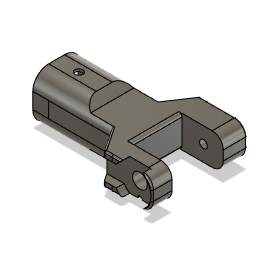
SholderFork_1 v20 (Autodesk Fusion 360 design; units mm, degrees)
Autodesk Fusion 360 part; units mm, degrees
note: some values were not read from the file. Chosen so that the rebuilt part matches the saved one: which face or edge a step refers to. Set by a fixed rule: which sketch regions a step uses.
sketch "Sketch1" plane through (0, 0, 0) normal (0, 1, 0) x (1, 0, 0)
  line L0 (-50, -15) -> (-10, -15)
  line L1 (-50, 15) -> (-10, 15)
  line L2 (5, -15) -> (5, 15)
  line L3 (30, 30) -> (5, 30)
  line L4 (30, -30) -> (5, -30)
  line L5 (5, -15) -> (30, -15)
  line L6 (30, -15) -> (30, -30)
  line L7 (5, 15) -> (30, 15)
  line L8 (30, 15) -> (30, 30)
  line L9 (-10, -15) -> (0, -30)
  line L10 (0, -30) -> (5, -30)
  line L11 (-10, 15) -> (0, 30)
  line L12 (0, 30) -> (5, 30)
  line L13 (-10, 15) -> (-10, -15)
  line L14 (-50, 15) -> (-60, 15)
  line L15 (-60, 15) -> (-60, -15)
  line L16 (-60, -15) -> (-50, -15)
  constraint horizontal L3
  constraint perpendicular L2 L5
  constraint perpendicular L4 L6
  constraint perpendicular L2 L7
  constraint perpendicular L3 L8
  constraint perpendicular L0 L13
  constraint perpendicular L14 L15
extrude "Extrude1" add sketch "Sketch1" along normal blind 30 makes body 1
sketch "Sketch3" plane through (-60, 0, 0) normal (-1, 0, 0) x (0, 0, 1)
  line L0 (-15, 0) -> (15, 0)
  line L1 (15, 0) -> (15, 30)
  line L2 (15, 30) -> (-15, 30)
  line L3 (-15, 30) -> (-15, 0)
  circle A0 through (13.6, 15, 10) (-6.8, 26.7779, 10) (-6.8, 3.2221, 10)
  line L4 (-15, 0) -> (15, 0)
  line L5 (15, 0) -> (15, 30)
  line L6 (15, 30) -> (-15, 30)
  line L7 (-15, 30) -> (-15, 0)
  dimension "d64" = 27.2
sketch "Sketch3 (curves 10 mm off its plane)" plane through (-70, 0, 0) normal (-1, 0, 0) x (0, 0, 1)
  circle A0 centre (0, 15) radius 13.6
extrude "Extrude3" cut sketch "Sketch3 (curves 10 mm off its plane)" against normal blind 36 bodies 1
sketch "Sketch4" plane through (0, 30, 0) normal (0, 1, 0) x (-1, 0, 0)
  line L0 (50, 15) -> (10, 15)
  line L1 (10, 15) -> (0, 30)
  line L2 (0, 30) -> (-5, 30)
  line L3 (-5, 30) -> (-30, 30)
  line L4 (-30, 30) -> (-30, 15)
  line L5 (-30, 15) -> (-5, 15)
  line L6 (-5, 15) -> (-5, -15)
  line L7 (-5, -15) -> (-30, -15)
  line L8 (-30, -15) -> (-30, -30)
  line L9 (-30, -30) -> (-5, -30)
  line L10 (-5, -30) -> (0, -30)
  line L11 (0, -30) -> (10, -15)
  line L12 (10, -15) -> (60, -15)
  line L13 (25, -10) -> (25, -15)
  line L14 (25, -10) -> (25, 15)
  line L15 (60, -15) -> (60, 15)
  line L16 (60, 15) -> (50, 15)
  constraint coincident L12 L13.end
  constraint perpendicular L12 L13
  constraint coincident L0 L14.end
  constraint perpendicular L0 L14
extrude "Extrude4" cut sketch "Sketch4" against normal blind 5 contours L0 L1 L2 L3 L4 L5 L6 L7 L8 L9 L10 L11 L12 L13 L14 bodies 1
sketch "Sketch5" plane through (0, 0, 0) normal (0, -1, 0) x (1, 0, 0)
  line L0 (-60, -15) -> (-10, -15)
  line L1 (-10, -15) -> (0, -30)
  line L2 (0, -30) -> (5, -30)
  line L3 (5, -30) -> (30, -30)
  line L4 (30, -30) -> (30, -15)
  line L5 (30, -15) -> (5, -15)
  line L6 (5, -15) -> (5, 15)
  line L7 (5, 15) -> (30, 15)
  line L8 (30, 15) -> (30, 30)
  line L9 (30, 30) -> (5, 30)
  line L10 (5, 30) -> (0, 30)
  line L11 (0, 30) -> (-10, 15)
  line L12 (-10, 15) -> (-50, 15)
  line L13 (-25, 14) -> (-25, 15)
  line L14 (-25, 14) -> (-25, -15)
  line L15 (-50, 15) -> (-60, 15)
  line L16 (-60, 15) -> (-60, -15)
  constraint coincident L12 L13.end
  constraint perpendicular L12 L13
  constraint perpendicular L12 L14
extrude "Extrude5" cut sketch "Sketch5" against normal blind 5 contours L0 L1 L2 L3 L4 L5 L6 L7 L8 L9 L10 L11 L12 L13 L14 bodies 1
chamfer "Chamfer1" distance 5 angle 45 2 edges at (-25, 0, 0) (-25, 30, 0) on bodies 1
fillet "Fillet2" radius 10 4 edges at (-45, 30, -15) (-40, 30, 15) (-40, 0, 15) (-45, 0, -15) on bodies 1
sketch "Sketch2" plane through (0, 0, 30) normal (0, 0, 1) x (1, 0, 0)
  line L0 (30, 5) -> (30, 25)
  line L1 (5, 25) -> (5, 5)
  line L2 (5, 5) -> (30, 5)
  line L3 (30, 25) -> (5, 25)
  line L4 (11.0494, 5) -> (23.9506, 5)
  arc A0 (23.9506, 5) -> (23.9506, 25) centre (17.5, 15) ccw
  arc A1 (19, 5) -> (16, 5) centre (17.5, 5) ccw
  line L5 (5.6, 8.5) -> (7.5321, 8.5)
  line L6 (5.6, 21.5) -> (7.5321, 21.5)
  line L7 (5.6, 21.5) -> (5, 21.5)
  line L8 (5.6, 8.5) -> (5, 8.5)
  arc A2 (11.0494, 25) -> (7.5321, 21.5) centre (17.5, 15) ccw
  arc A3 (7.5321, 8.5) -> (11.0494, 5) centre (17.5, 15) ccw
  line L9 (5, 21.5) -> (-2, 21.5)
  line L10 (5, 8.5) -> (-2, 8.5)
  line L11 (-2, 8.5) -> (-4, 8.5)
  line L12 (-4, 8.5) -> (-4, 21.5)
  line L13 (-2, 21.5) -> (-4, 21.5)
  circle A4 centre (17.5, 15) radius 4.65
  dimension "d65" = 23.8
  dimension "d69" = 9.3
  constraint coincident L3 A0.end
  constraint coincident L3 A2.start
  constraint coincident L2 L4.end
  constraint concentric A0 A2
  constraint coincident L2 A1.end
  constraint coincident L2 A1.start
  constraint coincident L5.end A2
  constraint coincident L1 L7.end
  constraint perpendicular L1 L7
  constraint coincident L1 L8.end
  constraint perpendicular L1 L8
  constraint concentric A2 A3
  constraint perpendicular L1 L9
  constraint perpendicular L10 L12
  constraint perpendicular L12 L13
  measures "d65" diameter of A2
  measures "d69" diameter of A4
extrude "Extrude6" cut sketch "Sketch2" against normal blind 5 contours L1 L2 L3 L4 A0 A1 L5 L6 L7 L8 A2 A3 | L1 L9 L10 L11 L12 L13 | A4 bodies 1
copy_body "Body->Comp1" bodies 1 removing the originals makes body 2 in component "Component"
fillet "Fillet2'" radius 2 2 edges at (5, 25, 0) (5, 5, 0) on bodies 2 in component "Component"
extrude "Extrude1'" cut sketch "Sketch2" against normal blind 16 contours A4 bodies 2 in component "Component"
sketch "Sketch6" plane through (0, 0, -30) normal (0, 0, -1) x (-1, 0, 0)
  line L0 (-30, 5) -> (-5, 5)
  line L1 (-5, 5) -> (-5, 25)
  line L2 (-5, 25) -> (-30, 25)
  line L3 (-30, 25) -> (-30, 5)
  circle A0 centre (-17.5, 15) radius 2.45
  point P0 (-17.5, 15)
  dimension "d33" = 4.9
  constraint coincident P0 A0.centre
  measures "d33" diameter of A0
extrude "Extrude5'" cut sketch "Sketch6" against normal blind 16 contours A0 bodies 2 in component "Component"
sketch "Sketch7" plane through (0, 0, -30) normal (0, 0, -1) x (-1, 0, 0)
  circle A0 centre (-17.5, 15) radius 2.45
  line L0 (-30, 5) -> (-5, 5)
  line L1 (-5, 5) -> (-5, 25)
  line L2 (-5, 25) -> (-30, 25)
  line L3 (-30, 25) -> (-30, 5)
  line L4 (-13.6, 15) -> (-13.6, 17.2517)
  line L5 (-13.6, 15) -> (-13.6, 12.7483)
  line L6 (-15.55, 18.3775) -> (-17.5, 19.5033)
  line L7 (-15.55, 18.3775) -> (-13.6, 17.2517)
  line L8 (-19.45, 18.3775) -> (-21.4, 17.2517)
  line L9 (-19.45, 18.3775) -> (-17.5, 19.5033)
  line L10 (-21.4, 15) -> (-21.4, 12.7483)
  line L11 (-21.4, 15) -> (-21.4, 17.2517)
  line L12 (-19.45, 11.6225) -> (-17.5, 10.4967)
  line L13 (-19.45, 11.6225) -> (-21.4, 12.7483)
  line L14 (-15.55, 11.6225) -> (-13.6, 12.7483)
  line L15 (-15.55, 11.6225) -> (-17.5, 10.4967)
  dimension "d40" = 3.9
  measures "d40" distance of A0.centre L4.start
extrude "Extrude6'" cut sketch "Sketch7" against normal blind 5 contours L4 L5 L6 L7 L8 L9 L10 L11 L12 L13 L14 L15 bodies 2 in component "Component"
fillet "Fillet3" radius 7 4 edges at (30, 25, 22.5) (30, 25, -22.5) (30, 5, 22.5) (30, 5, -22.5) on bodies 2 in component "Component"
move_face "OffsetFaces1" offset -2.25 1 faces at (7.6167, 15, 15) on bodies 2 in component "Component"
sketch "Sketch10" plane through (0, 30, 0) normal (0, 1, 0) x (-1, 0, 0)
  line L0 (60, 5) -> (30, 5)
  line L1 (30, -5) -> (60, -5)
  circle A0 centre (46, -0.0923) radius 2.5
  line L2 (30, 5) -> (30, -5)
  line L3 (60, -5) -> (60, 5)
  dimension "d58" = 5
  measures "d58" diameter of A0
extrude "Extrude8" cut sketch "Sketch10" against normal blind 32 contours A0 bodies 2 in component "Component"
fillet "Fillet4" radius 1 21 edges at (2.5, 25, -30) (14, 25, -30) (27.9497, 22.9497, -30) (30, 15, -30) (27.9497, 7.0503, -30) (14, 5, -30) (2.5, 5, -30) (-5.4466, 25, -21.8301) (-5.4466, 5, -21.8301) (8.0247, 25, 30) (2.5, 25, 30) (-5.4466, 25, 21.8301) (2.5, 5, 30) (8.0247, 5, 30) (-5.4466, 5, 21.8301) (0, 6.75, 30) (0, 23.25, 30) (0, 15, -30) (28.3173, 22.5526, 30) (30, 15, 30) (28.3173, 7.4474, 30) on bodies 2 in component "Component"
extrude "Extrude9" cut 1 faces at (17.3887, 5.4875, 30) along direction (0, 0, -1) blind 9 on bodies 2 bodies 2 in component "Component"
move_face "OffsetFaces2" offset -1 1 faces at (5, 17.6667, 6.5) on bodies 2 in component "Component"
component "Component" placed x (1, 0, 0) y (0, 1, 0) z (0, 0, 1) at (0, 0, 0)
